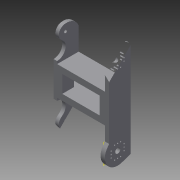
# Autodesk Inventor part: cadera
Saved by Autodesk Inventor 2015 (Build 190159000, 159)
## iProperties
Created: 2015-08-01
Part Number: cadera
Material: Genérico
Document SubType Name: Modeling
Designer: Roberto
Density: 1 g/cm^3
Appearance: Valor por defecto
Author: Roberto
Autodesk Inventor part; units mm, degrees
ref_plane "YZ Plane" through (0, 0, 0) normal (1, 0, 0) x (0, 1, 0)
ref_plane "XZ Plane" through (0, 0, 0) normal (0, 1, 0) x (-1, 0, 0)
ref_plane "XY Plane" through (0, 0, 0) normal (0, 0, 1) x (1, 0, 0)
ref_plane "Plano de trabajo1" through (129.4922, 102.1402, -54.3752) normal (1, 0, 0) x (0, 1, 0)
sketch "Boceto1" plane through (129.4922, 102.1402, -54.3752) normal (1, 0, 0) x (0, 1, 0)
  circle A0 centre (-7.5, 0) radius 0.75 projected
  circle A1 centre (3.5, 7.5) radius 0.75 projected
  circle A2 centre (-3.5, 7.5) radius 0.75 projected
  circle A3 centre (7.5, 0) radius 0.75 projected
  circle A4 centre (-3.5, -7.5) radius 0.75 projected
  circle A5 centre (0, -7.5) radius 0.75 projected
  circle A6 centre (3.5, -7.5) radius 0.75 projected
  circle A7 centre (7.5, 3.5) radius 0.75 projected
  circle A8 centre (7.5, -3.5) radius 0.75 projected
  circle A9 centre (0, 7.5) radius 0.75 projected
  circle A10 centre (-7.5, -3.5) radius 0.75 projected
  circle A11 centre (-7.5, 3.5) radius 0.75 projected
  circle A12 centre (0, 0) radius 3 projected
  circle A13 centre (0, 0) radius 10.5 projected
  arc A14 (-12.2873, 8.6036) -> (5.1303, -14.0954) centre (0, 0) ccw
  line L0 (-12.2873, 8.6036) -> (-10, 11.8702)
  line L1 (-10, 11.8702) -> (-10, 45)
  line L2 (-10, 45) -> (15, 45)
  line L3 (15, 45) -> (15, -10.5031)
  line L4 (15, -10.5031) -> (5.1303, -14.0954)
  point P0 (-102.1402, 54.3752)
  dimension "d0" = 15
  dimension "d1" = 45
  dimension "d2" = 10
  dimension "d3" = 25
  dimension "d4" = 145
  dimension "d5" = 70
  constraints: 10 end point, 3 point on circle, 2 perpendicular, 2 tangent, 1 centre point, 1 coincident, 1 vertical
  measures "d0" radius of A14
  measures "d1" distance from line of A12.centre L2
  measures "d2" distance from line of A12.centre L1
  measures "d3" distance of L1.end L2.end
  measures "d4" angle of L1 L0
  measures "d5" angle of L4 L3
extrude "Extrusión1" add sketch "Boceto1" along normal blind 5 contours A13 | L0 L1 L2 L3 L4 A14
sketch "Boceto2" plane through (129.4922, 102.1402, -54.3752) normal (-1, 0, 0) x (0, 0, 1)
  line L0 (35, -10) -> (28, -10)
  line L1 (28, -10) -> (28, 15)
  line L2 (28, 15) -> (35, 15)
  line L3 (35, 15) -> (35, -10)
  line L4 (45, -10) -> (11.8702, -10) projected
  line L5 (-10.5031, 15) -> (45, 15) projected
  line L6 (45, 15) -> (45, -10) projected
  point P0 (54.3752, -102.1402)
  dimension "d8" = 10
  dimension "d9" = 7
  constraints: 8 end point, 2 collinear, 2 parallel, 1 horizontal, 1 perpendicular
  measures "d8" distance between parallel lines of L6 L3
  measures "d9" distance of L1.end L2.end
extrude "Extrusión2" add sketch "Boceto2" along normal blind 55.5 contours L0 L1 L2 L3
sketch "Boceto4" plane through (73.9922, 102.1402, -54.3752) normal (-1, 0, 0) x (0, 0, 1)
  line L0 (35, 15) -> (28, 15) projected
  line L1 (35, 15) -> (45, 15) projected
  line L2 (45, 15) -> (45, -10) projected
  line L3 (45, -10) -> (35, -10) projected
  line L4 (28, -10) -> (35, -10) projected
  line L5 (-10.5031, 15) -> (28, 15) projected
  circle A0 centre (0, 0) radius 1.8 projected
  line L6 (-10.5031, 15) -> (45, 15) projected
  arc A1 (-7.9151, -1.1622) -> (6.6543, -4.4407) centre (0, 0) ccw
  arc A2 (1.4969, 15) -> (-7.9151, -1.1622) centre (6.9257, 1.0169) ccw
  line L7 (28, -10) -> (25, -10)
  arc A3 (25, -10) -> (6.6543, -4.4407) centre (14.9848, -10) ccw
  point P0 (54.3752, -102.1402)
  dimension "d20" = 8
  dimension "d21" = 12
  dimension "d23" = 15
  dimension "d24" = 20
  constraints: 6 point on circle, 3 centre point, 2 end point, 2 tangent, 1 collinear, 1 concentric, 1 line through centre, 1 point on line
  measures "d20" radius of A1
  measures "d21" distance of L5.start A2.start
  measures "d23" radius of A2
  measures "d24" distance of L2.end L7.end
extrude "Extrusión4" add sketch "Boceto4" along normal blind 4
sketch "Boceto7" plane through (134.4922, 102.1402, -54.3752) normal (1, 0, 0) x (0, 0, -1)
  line L0 (-45, 15) -> (-45, -10) projected
  line L1 (10.5031, 15) -> (-45, 15) projected
  point P0 (-54.3752, -102.1402)
  point P1 (-24, 7)
  point P2 (-40, 12)
  dimension "d38" = 21
  dimension "d39" = 8
  dimension "d47" = 3
  dimension "d48" = 5
  measures "d38" distance from line of L0 point (-24, 7)
  measures "d39" distance from line of L1 point (-24, 7)
  measures "d47" distance from line of L1 point (-40, 12)
  measures "d48" distance from line of L0 point (-40, 12)
hole "Agujero2" at (134.4922, 109.1402, -30.3752) at (134.4922, 114.1402, -14.3752) direction (-1, 0, 0) diameter 2.5 end through all
mirror "Simetría1" about plane through (73.9922, 92.1402, -9.3752) normal (0, 0, 1)
sketch "Boceto5" plane through (129.4922, 92.1402, -42.505) normal (0, -1, 0) x (1, 0, 0)
  line L0 (0, 43.1298) -> (-6, 43.1298)
  line L1 (-6, 43.1298) -> (-6, 23.1298)
  line L2 (-6, 23.1298) -> (0, 23.1298)
  line L3 (0, 23.1298) -> (0, 43.1298)
  line L4 (-55.5, 43.1298) -> (-49.5, 43.1298)
  line L5 (-49.5, 43.1298) -> (-49.5, 23.1298)
  line L6 (-49.5, 23.1298) -> (-55.5, 23.1298)
  line L7 (-55.5, 23.1298) -> (-55.5, 43.1298)
  point P0 (-129.4922, 42.505)
  dimension "d27" = 6
  constraints: 16 end point, 4 coincident, 4 parallel, 2 horizontal, 2 perpendicular, 1 collinear
  measures "d27" distance of L4.start L4.end
extrude "Extrusión5" add sketch "Boceto5" against normal blind 12
sketch "Boceto6" plane through (129.4922, 104.1402, -42.505) normal (0, 1, 0) x (1, 0, 0)
  circle A0 centre (-2.6, -28.2798) radius 2.2 projected
  circle A1 centre (-2.6, -38.0798) radius 2.2 projected
  circle A2 centre (-53, -28.2798) radius 2.2 projected
  circle A3 centre (-53, -38.0798) radius 2.2 projected
  point P0 (-129.4922, -42.505)
  constraints: 4 coincident
hole "Agujero1" at (126.8922, 104.1402, -14.2252) at (126.8922, 104.1402, -4.4252) at (76.4922, 104.1402, -14.2252) at (76.4922, 104.1402, -4.4252) direction (0, -1, 0) diameter 2.5 end through all
fillet "Empalme1" radius 2 4 edges at (73.9922, 104.6402, 7.6248) (73.9922, 104.6402, -26.3752) (129.4922, 104.6402, -26.3752) (129.4922, 104.6402, 7.6248)
fillet "Empalme2" radius 5 2 edges at (131.9922, 92.1402, 23.7546) (131.9922, 92.1402, -42.505)
fillet "Empalme3" radius 3 2 edges at (71.9922, 92.1402, 10.6248) (71.9922, 92.1402, -29.3752)
